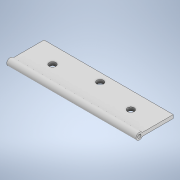
# Autodesk Inventor part: hinge
Saved by Autodesk Inventor 2021.5 (Build 255421000, 421)
## iProperties
Created: 2024-11-18
Part Number: hinge
Material: Generic
Document SubType Name: Modeling
Designer: email
Density: 1 g/cm^3
Appearance: Default
Author: email
Autodesk Inventor part; units mm, degrees
ref_plane "YZ Plane" through (0, 0, 0) normal (1, 0, 0) x (0, 1, 0)
ref_plane "XZ Plane" through (0, 0, 0) normal (0, 1, 0) x (-1, 0, 0)
ref_plane "XY Plane" through (0, 0, 0) normal (0, 0, 1) x (1, 0, 0)
sketch "Sketch1" plane through (0, 0, 0) normal (0, 1, 0) x (-1, 0, 0)
  line L0 (0, 0) -> (-76.2, 0)
  line L1 (-76.2, 0) -> (-76.2, -20)
  line L2 (-76.2, -20) -> (0, -20)
  line L3 (0, -20) -> (0, 0)
  line L4 (0, 0) -> (-76.2, 0)
  line L5 (-76.2, 0) -> (-76.2, -10)
  line L6 (-76.2, -10) -> (0, -10) construction
  line L7 (0, -10) -> (0, 0)
  line L8 (0, -10) -> (-15, -10)
  line L9 (-76.2, -10) -> (-61.2, -10)
  line L10 (-38.1, -10) -> (-38.1, -15)
  dimension "d0" = 20
  dimension "d1" = 76.2
  dimension "d2" = 10
  dimension "d3" = 15
  dimension "d4" = 15
  dimension "d5" = 5
  constraints: 22 end point, 4 parallel, 2 horizontal, 2 midpoint, 2 perpendicular, 2 point on line, 1 vertical
  measures "d0" distance of L0.end L1.end
  measures "d1" distance of L1.end L2.end
  measures "d2" distance between parallel lines of L0 L6
  measures "d3" distance of L6.end L8.end
  measures "d4" distance from line of L1 L9.end
  measures "d5" distance of L10.start L10.end
extrude "Extrusion1" add sketch "Sketch1" along normal blind 2
hole "Hole1" at (15, 0, -10) at (38.1, 0, -15) at (61.2, 0, -10) direction (0, 1, 0) diameter 4 depth 10 tip angle 118
sketch "Sketch2" plane through (76.2, 0, 0) normal (1, 0, 0) x (0, 0, -1)
  line L0 (0, 0) -> (0, 1)
  circle A0 centre (0, 1) radius 2
  circle A1 centre (0, 1) radius 1
  dimension "d15" = 1
  dimension "d16" = 4
  dimension "d19" = 2
  constraints: 2 centre point, 2 coincident, 2 end point, 1 vertical
  measures "d15" distance of L0.start L0.end
  measures "d16" diameter of A0
  measures "d19" diameter of A1
extrude "Extrusion2" add sketch "Sketch2" against normal blind 76.2
extrude "Extrusion4" cut sketch "Sketch2" against normal blind 76.2 contours A1
body "Solid1"
